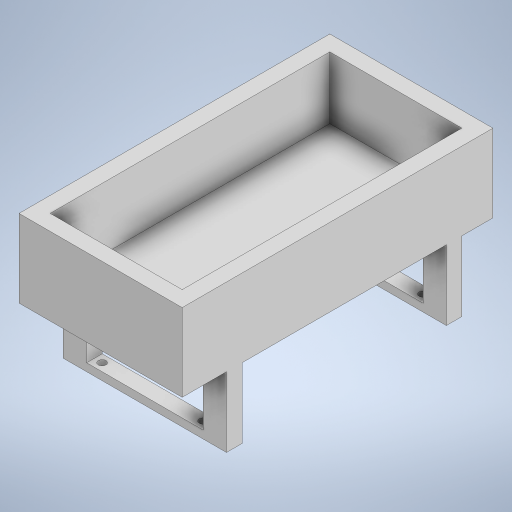
# Autodesk Inventor part: container
Saved by Autodesk Inventor 2023 (Build 270158000, 158)
## iProperties
Created: 2022-07-03
Part Number: container
Material: Genérico
Document SubType Name: Modeling
Designer: inigo
Density: 1 g/cm^3
Appearance: Valor por defecto
Author: inigo
Autodesk Inventor part; units mm, degrees
ref_plane "YZ Plane" through (0, 0, 0) normal (1, 0, 0) x (0, 1, 0)
ref_plane "XZ Plane" through (0, 0, 0) normal (0, 1, 0) x (-1, 0, 0)
ref_plane "XY Plane" through (0, 0, 0) normal (0, 0, 1) x (1, 0, 0)
sketch "Boceto1" plane through (0, 0, 0) normal (0, 1, 0) x (-1, 0, 0)
  line L0 (105, 200) -> (-105, 200)
  line L1 (-105, 200) -> (-105, -200)
  line L2 (-105, -200) -> (105, -200)
  line L3 (105, -200) -> (105, 200)
  line L4 (105, 200) -> (-105, -200) construction
  line L5 (-105, 200) -> (105, -200) construction
  point P0 (0, 0)
  dimension "d0" = 210
  dimension "d1" = 400
  constraints: 12 end point, 2 midpoint, 2 parallel, 1 horizontal, 1 perpendicular
  measures "d0" distance of L2.end L1.end
  measures "d1" distance of L1.end L0.end
extrude "Extrusión1" add sketch "Boceto1" along normal blind 100
sketch "Boceto2" plane through (0, 100, 0) normal (0, 1, 0) x (1, 0, 0)
  line L0 (-85, -180) -> (85, -180)
  line L1 (85, -180) -> (85, 180)
  line L2 (85, 180) -> (-85, 180)
  line L3 (-85, 180) -> (-85, -180)
  line L4 (-85, -180) -> (85, 180) construction
  line L5 (85, -180) -> (-85, 180) construction
  point P0 (0, 0)
  dimension "d4" = 170
  dimension "d5" = 360
  constraints: 12 end point, 2 midpoint, 2 parallel, 1 horizontal, 1 perpendicular
  measures "d4" distance of L2.end L1.end
  measures "d5" distance of L1.end L0.end
extrude "Extrusión2" cut sketch "Boceto2" against normal blind 80
sketch "Boceto3" plane through (0, 0, 0) normal (0, -1, 0) x (1, 0, 0)
  line L0 (105, 143) -> (75, 143)
  line L1 (75, 143) -> (75, 123)
  line L2 (75, 123) -> (105, 123)
  line L3 (105, 123) -> (105, 143)
  line L4 (105, 143) -> (75, 123) construction
  line L5 (75, 143) -> (105, 123) construction
  line L6 (105, -140) -> (75, -140)
  line L7 (75, -140) -> (75, -160)
  line L8 (75, -160) -> (105, -160)
  line L9 (105, -160) -> (105, -140)
  line L10 (105, -140) -> (75, -160) construction
  line L11 (75, -140) -> (105, -160) construction
  line L12 (105, -200) -> (-105, -200) projected
  line L13 (-105, 143) -> (-75, 143)
  line L14 (-75, 143) -> (-75, 123)
  line L15 (-75, 123) -> (-105, 123)
  line L16 (-105, 123) -> (-105, 143)
  line L17 (-105, 143) -> (-75, 123) construction
  line L18 (-75, 143) -> (-105, 123) construction
  line L19 (-105, -140) -> (-75, -140)
  line L20 (-75, -140) -> (-75, -160)
  line L21 (-75, -160) -> (-105, -160)
  line L22 (-105, -160) -> (-105, -140)
  line L23 (-105, -140) -> (-75, -160) construction
  line L24 (-75, -140) -> (-105, -160) construction
  line L25 (-105, 200) -> (105, 200) projected
  point P0 (0, 0)
  point P1 (90, 133)
  point P2 (105, 133)
  point P3 (90, -150)
  point P4 (105, -150)
  point P5 (-90, 35)
  point P6 (-105, 35)
  point P7 (-90, -150)
  point P8 (-105, -150)
  point P9 (-90, 143)
  dimension "d9" = 20
  dimension "d12" = 20
  dimension "d34" = 57
  dimension "d35" = 57
  dimension "d36" = 20
  dimension "d37" = 40
  dimension "d38" = 40
  constraints: 44 end point, 7 midpoint, 4 parallel, 2 horizontal, 2 perpendicular, 6 other
  measures "d9" distance of L1.end L0.end
  measures "d12" distance of L7.end L6.end
  measures "d34" distance between parallel lines of L0 L25
  measures "d35" distance between parallel lines of L25 L13
  measures "d36" distance from line of L15 point (-90, 143)
  measures "d37" distance between parallel lines of L12 L21
  measures "d38" distance between parallel lines of L12 L8
extrude "Extrusión3" add sketch "Boceto3" along normal blind 90
sketch "Boceto6" plane through (-75, 0, 143) normal (1, 0, 0) x (0, 0, -1)
  line L0 (0, 0) -> (0, -90) projected
  line L1 (20, 0) -> (20, -90) projected
  line L2 (0, -90) -> (20, -90)
  line L3 (20, -90) -> (20, -80)
  line L4 (20, -80) -> (0, -80)
  line L5 (0, -80) -> (0, -90)
  point P0 (143, 0)
  dimension "d16" = 10
  constraints: 8 end point, 2 parallel, 1 horizontal, 1 perpendicular, 1 point on line
  measures "d16" distance of L3.end L2.end
extrude "Extrusión4" add sketch "Boceto6" along normal blind 150
sketch "Boceto7" plane through (-75, 0, -140) normal (1, 0, 0) x (0, 0, -1)
  line L0 (0, 0) -> (0, -90) projected
  line L1 (20, 0) -> (20, -90) projected
  line L2 (0, -90) -> (20, -90)
  line L3 (20, -90) -> (20, -80)
  line L4 (20, -80) -> (0, -80)
  line L5 (0, -80) -> (0, -90)
  point P0 (-140, 0)
  dimension "d19" = 10
  constraints: 8 end point, 2 parallel, 1 horizontal, 1 perpendicular, 1 point on line
  measures "d19" distance of L3.end L2.end
extrude "Extrusión5" add sketch "Boceto7" along normal blind 150
sketch "Boceto8" plane through (0, -90, 0) normal (0, -1, 0) x (1, 0, 0)
  circle A0 centre (-65, 133) radius 5
  circle A1 centre (65, 133) radius 5
  line L0 (-105, 143) -> (-105, 123) projected
  line L1 (105, 123) -> (105, 143) projected
  line L2 (60, 123) -> (60, 143)
  line L3 (105, 143) -> (-105, 143) projected
  point P0 (0, 0)
  dimension "d22" = 10
  dimension "d23" = 10
  dimension "d24" = 40
  dimension "d25" = 40
  dimension "d39" = 10
  dimension "d40" = 10
  constraints: 2 centre point, 2 end point, 1 vertical
  measures "d22" diameter of A0
  measures "d23" diameter of A1
  measures "d24" distance from line of L0 A0.centre
  measures "d25" distance from line of A1.centre L1
  measures "d39" distance from line of L3 A1.centre
  measures "d40" distance from line of L3 A0.centre
sketch "Boceto9" plane through (0, -90, 0) normal (0, -1, 0) x (1, 0, 0)
  circle A0 centre (-65, -150) radius 5
  circle A1 centre (65, -150) radius 5
  line L0 (-105, -140) -> (-105, -160) projected
  line L1 (105, -160) -> (105, -140) projected
  point P0 (0, 0)
  dimension "d26" = 10
  dimension "d27" = 10
  dimension "d28" = 40
  dimension "d29" = 40
  constraints: 2 centre point
  measures "d26" diameter of A0
  measures "d27" diameter of A1
  measures "d28" distance from line of L0 A0.centre
  measures "d29" distance from line of L1 A1.centre
extrude "Extrusión6" cut sketch "Boceto8" against normal blind 20
extrude "Extrusión7" cut sketch "Boceto9" against normal blind 20
